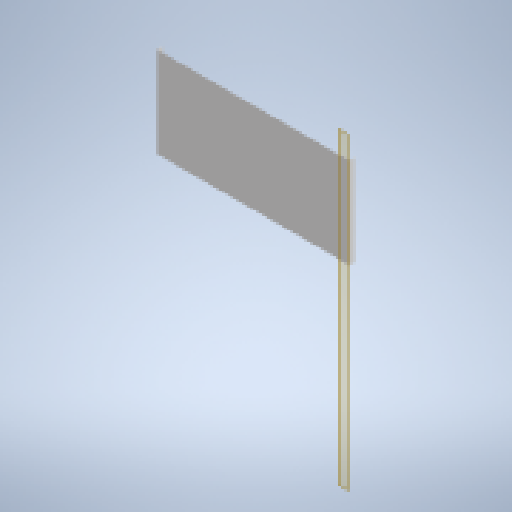
# Autodesk Inventor part: ENGINE_BASE
Saved by Autodesk Inventor 2024 (Build 280153000, 153)
## iProperties
Created: 2024-04-11
Part Number: ENGINE_BASE
Material: Generic
Document SubType Name: Sheet Metal
Designer: teeta
Density: 1 g/cm^3
Sheet Metal Rule: Default_mm
Appearance: Default
Author: teeta
Autodesk Inventor part; units mm, degrees
ref_plane "YZ Plane" through (0, 0, 0) normal (1, 0, 0) x (0, 1, 0)
ref_plane "XZ Plane" through (0, 0, 0) normal (0, 1, 0) x (-1, 0, 0)
ref_plane "XY Plane" through (0, 0, 0) normal (0, 0, 1) x (1, 0, 0)
ref_plane "Work Plane1" through (0, 0, 0) normal (0, 0, 1) x (1, 0, 0)
sketch "Sketch1" plane through (0, 0, 0) normal (0, 0, 1) x (1, 0, 0)
  line L0 (-849.45, 463.2386) -> (11.35, 463.2386)
  line L1 (11.35, 463.2386) -> (11.35, 863.2386)
  line L2 (11.35, 863.2386) -> (-849.45, 863.2386)
  line L3 (-849.45, 863.2386) -> (-849.45, 463.2386)
  line L4 (-844.45, 1225.4) -> (-844.45, -25.4)
  line L5 (6.35, -25.4) -> (6.35, 1225.4)
  point P0 (0, 0)
  point P1 (6.35, 463.2386)
  point P2 (6.35, 863.2386)
  point P3 (-844.45, 863.2386)
  point P4 (-844.45, 463.2386)
  dimension "d1" = 400
  dimension "d2" = 5
  dimension "d3" = 5
  measures "d1" distance of L2.end L0.start
  measures "d2" distance between parallel lines of L4 L3
  measures "d3" distance between parallel lines of L5 L1
extrude "Plate1" add sketch "Sketch1" along normal blind 0.5 contours L4 L2 L5 L0
sketch "Sketch2" plane through (5.85, 863.2386, 0.5) normal (1, 0, 0) x (0, 1, 0)
  line L0 (-400, 0) -> (0, 0)
  line L1 (0, 0) -> (0, 25)
  line L2 (0, 25) -> (-400, 25)
  line L3 (-400, 25) -> (-400, 0)
  constraints: 6 end point, 1 horizontal, 1 perpendicular, 1 vertical
edge flange "Flange1" height 25 angle 90 thickness 0.5 bend radius 0.5 thickness toward (1, 0, 0) relief straight relief width 0.5 relief depth 0.25 corner gap 0.5 corner form 0 edges at (6.35, 663.2386, 0.5) (-844.45, 663.2386, 0.5) wall of the first edge with corners at (5.85, 463.2386, 0.5) (5.85, 863.2386, 0.5) (5.85, 863.2386, -24.5) (5.85, 463.2386, -24.5)
bend "Bend1"
corner "Corner1"
move faces "Move1" translate (0, 320.75, 0) faces at (-560.5167, 463.2386, 0.3333) (-277.5833, 863.2386, 0.3333)
equation "\"d4\" = Thickness"
equation "\"d5\" = BendReliefWidth"
equation "\"d6\" = BendReliefDepth"
equation "\"d7\" = MinimumRemnant"
equation "\"d8\" = TransitionRadius"
equation "\"d11\" = BendRadius"
equation "\"d12\" = CornerReliefSize"
equation "\"d13\" = GapSize"
equation "\"d14\" = JacobiRadiusSize"
equation "\"BendRadius\" = Thickness"
equation "\"BendReliefWidth\" = Thickness"
equation "\"BendReliefDepth\" = 0.5 * Thickness"
equation "\"CornerReliefSize\" = 4 * Thickness"
equation "\"MinimumRemnant\" = 2 * Thickness"
equation "\"TransitionRadius\" = BendRadius"
equation "\"JacobiRadiusSize\" = BendRadius"
equation "\"GapSize\" = Thickness"
equation "\"Thickness\" = 0.5"
body "Solid1"
